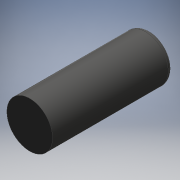
# Autodesk Inventor part: ES Helix Antenna
Saved by Autodesk Inventor 2016 SP1 (Build 200210100, 210)
## iProperties
Created: 2016-12-17
Part Number: ES Helix Antenna
Material: Rubber, Silicone
Document SubType Name: Modeling
Designer: eschr_000
Mass: 14 g
Surface Area: 33.2217 cm^2
Volume: 13.0701 cm^3
Density: 1.07115 g/cm^3
Appearance: Rubber - Black
Author: E.S. Schroen
Comments: Weight: 14 g Frequency: 1616-1626 MHz Polarization: RHCP Antenna element peak gain: 2.8 dBic (typical) Efficiency: 60% Bandwidth: (-1dB) 20 MHz Axial Ratio: 0.2 dB (typical) / 0.5 dB (max) VSWR: 1.5 (max) Impedance: 50 Ohm Operating temp.: from -40˚C to 85˚C RF connector: SMA
Autodesk Inventor part; units mm, degrees
ref_plane "YZ Plane" through (0, 0, 0) normal (1, 0, 0) x (0, 1, 0)
ref_plane "XZ Plane" through (0, 0, 0) normal (0, 1, 0) x (-1, 0, 0)
ref_plane "XY Plane" through (0, 0, 0) normal (0, 0, 1) x (1, 0, 0)
sketch "Sketch1" plane through (0, 0, 0) normal (0, 1, 0) x (-1, 0, 0)
  circle A0 centre (0, 0) radius 9.25
  dimension "d0" = 18.5
  constraints: 1 centre point, 1 coincident
  measures "d0" diameter of A0
extrude "Extrusion1" add sketch "Sketch1" along normal blind 48.8
fillet "Fillet1" radius 2 1 edges at (9.25, 48.8, 0)
body "Solid1"
